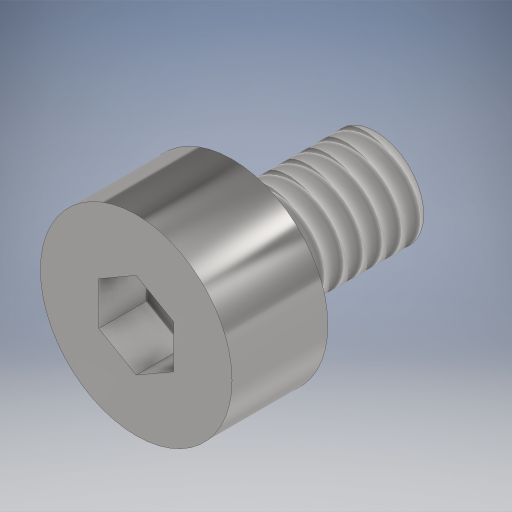
# Autodesk Inventor part: Болт М2
Saved by Autodesk Inventor 2023 (Build 270158000, 158)
## iProperties
Created: 2023-01-15
Part Number: Болт М2
Material: Типовые
Document SubType Name: Modeling
Designer: Admin
Density: 1 g/cm^3
Appearance: По умолчанию
Author: Admin
Autodesk Inventor part; units mm, degrees
ref_plane "YZ Plane" through (0, 0, 0) normal (1, 0, 0) x (0, 1, 0)
ref_plane "XZ Plane" through (0, 0, 0) normal (0, 1, 0) x (-1, 0, 0)
ref_plane "XY Plane" through (0, 0, 0) normal (0, 0, 1) x (1, 0, 0)
sketch "Эскиз1" plane through (0, 0, 0) normal (0, 0, 1) x (1, 0, 0)
  circle A0 centre (0, 0) radius 2
  circle A1 centre (0, 0) radius 1
  dimension "d0" = 4
  dimension "d1" = 2
  constraints: 2 centre point, 2 coincident
  measures "d0" diameter of A0
  measures "d1" diameter of A1
extrude "Выдавливание1" add sketch "Эскиз1" along normal blind 2 contours A0 | A1
extrude "Выдавливание2" add sketch "Эскиз1" against normal blind 3 contours A1
thread "Резьба1" size "M2x0.4" class "6g" standard "ISO Metric profile" full length
sketch "Эскиз2" plane through (0, 0, 2) normal (0, 0, 1) x (1, 0, 0)
  line L0 (0, 0.9007) -> (0.78, 0.4503)
  line L1 (0.78, 0.4503) -> (0.78, -0.4503)
  line L2 (0.78, -0.4503) -> (0, -0.9007)
  line L3 (0, -0.9007) -> (-0.78, -0.4503)
  line L4 (-0.78, -0.4503) -> (-0.78, 0.4503)
  line L5 (-0.78, 0.4503) -> (0, 0.9007)
  point P0 (0, 0)
  point P1 (0, 0)
  dimension "d8" = 1.56
  constraints: 12 end point, 1 coincident, 1 vertical, 13 other
  measures "d8" distance between parallel lines of L4 L1
extrude "Выдавливание3" cut sketch "Эскиз2" against normal blind 1
